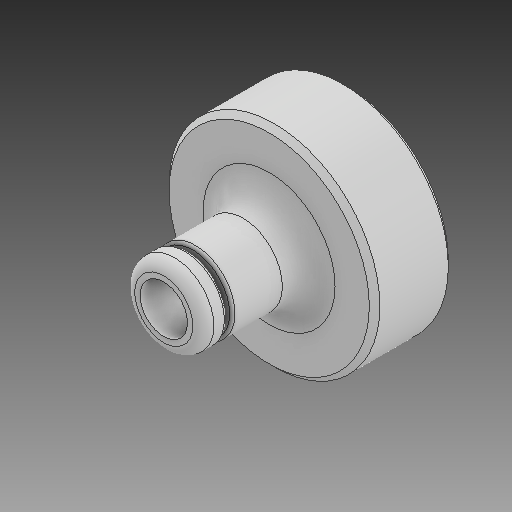
# Autodesk Inventor part: SchlauchAnschluss
Saved by Autodesk Inventor 2021 (Build 250183000, 183)
## iProperties
Created: 2021-11-19
Part Number: SchlauchAnschluss
Material: Generisch
Document SubType Name: Modeling
Designer: lukas
Density: 1 g/cm^3
Appearance: Vorgabe
Stock Number: Wasseranschluss
Author: lukas
Autodesk Inventor part; units mm, degrees
ref_plane "YZ Plane" through (0, 0, 0) normal (1, 0, 0) x (0, 1, 0)
ref_plane "XZ Plane" through (0, 0, 0) normal (0, 1, 0) x (-1, 0, 0)
sketch "Skizze1" plane through (0, 0, 0) normal (0, 0, 1) x (1, 0, 0)
  line L0 (-28, 0) -> (28, 0) projected
  line L1 (0, -28) -> (0, 28) projected
  circle A0 centre (0, 0) radius 20
  dimension "d0" = 40
  constraints: 1 centre point, 1 coincident
  measures "d0" diameter of A0
extrude "Extrusion1" add sketch "Skizze1" along normal blind 15
sketch "Skizze2" plane through (0, 0, 15) normal (0, 0, 1) x (1, 0, 0)
  circle A0 centre (0, 0) radius 7.5
  dimension "d3" = 15
  constraints: 1 centre point, 1 coincident
  measures "d3" diameter of A0
extrude "Extrusion2" add sketch "Skizze2" along normal blind 20
fillet "Rundung1" radius 5 1 edges at (-7.5, 0, 15)
chamfer "Fase1" distance 1 angle 45 2 edges at (-20, 0, 15) (-20, 0, 0)
fillet "Rundung2" radius 2 1 edges at (-7.5, 0, 35)
ref_plane "Arbeitsebene1" through (0, 0, 30) normal (0, 0, 1) x (1, 0, 0)
sketch "Skizze4" plane through (0, 0, 30) normal (0, 0, 1) x (1, 0, 0)
  circle A0 centre (0, 0) radius 5.5
  circle A1 centre (0, 0) radius 7.5
  constraints: 2 centre point, 2 coincident
extrude "Extrusion3" cut sketch "Skizze4" along normal mid plane 1
fillet "Rundung3" radius 0.5 2 edges at (-7.5, 0, 30.5) (-7.5, 0, 29.5)
sketch "Skizze5" plane through (0, 0, 35) normal (0, 0, 1) x (1, 0, 0)
  circle A0 centre (0, 0) radius 4.5
  dimension "d15" = 9
  constraints: 1 centre point, 1 coincident
  measures "d15" diameter of A0
extrude "Extrusion4" cut sketch "Skizze5" against normal blind 40
sketch "Skizze6" plane through (0, 0, 0) normal (0, 0, -1) x (-1, 0, 0)
  circle A0 centre (0, 0) radius 15
  dimension "d18" = 30
  constraints: 1 centre point, 1 coincident
  measures "d18" diameter of A0
extrude "Extrusion5" cut sketch "Skizze6" against normal blind 12
thread "Gewinde1" size "M30x3.5" class "6H" standard "ISO Metric profile" length 15
chamfer "Fase2" distance 1 angle 45 1 edges at (15, 0, 0)
chamfer "Fase3" distance 1 angle 45 1 edges at (-4.5, 0, 12)
